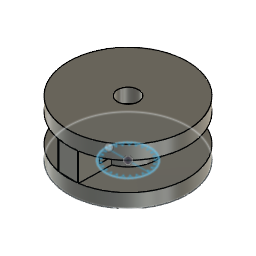
carrete servomotor (Autodesk Fusion 360 design; units mm, degrees)
part number: 2026-06-30-15-51-10-109
Autodesk Fusion 360 part; units mm, degrees
note: some values were not read from the file. Set by a fixed rule: which sketch regions a step uses.
sketch "Boceto1" plane through (0, 0, 0) normal (0, 0, 1) x (1, 0, 0)
  circle A0 centre (0, 0) radius 8.5
  line L0 (-3.15, 0) -> (3.15, 0)
  line L1 (-3.15, 0) -> (-2.6985, 0.2148)
  line L2 (-2.6985, 0.2148) -> (-3.1103, 0.4984)
  line L3 (-3.1103, 0.4984) -> (-3.15, 0)
  arc A1 (-3.15, 0) -> (-3.1103, 0.4984) centre (0, 0) ccw
  line L4 (-2.6672, -0.463) -> (-3.1366, -0.2907)
  line L5 (-3.1366, -0.2907) -> (-3.051, -0.7834)
  line L6 (-3.051, -0.7834) -> (-2.6672, -0.463)
  line L7 (-2.4682, -1.1117) -> (-2.9657, -1.0616)
  line L8 (-2.9657, -1.0616) -> (-2.7604, -1.5175)
  line L9 (-2.7604, -1.5175) -> (-2.4682, -1.1117)
  line L10 (-2.1142, -1.6906) -> (-2.6085, -1.7658)
  line L11 (-2.6085, -1.7658) -> (-2.2963, -2.1563)
  line L12 (-2.2963, -2.1563) -> (-2.1142, -1.6906)
  line L13 (-1.6273, -2.1633) -> (-2.0874, -2.3591)
  line L14 (-2.0874, -2.3591) -> (-1.6879, -2.6596)
  line L15 (-1.6879, -2.6596) -> (-1.6273, -2.1633)
  line L16 (-1.0382, -2.5) -> (-1.4352, -2.8041)
  line L17 (-1.4352, -2.8041) -> (-0.9734, -2.9958)
  line L18 (-0.9734, -2.9958) -> (-1.0382, -2.5)
  line L19 (-0.3839, -2.6797) -> (-0.6927, -3.0729)
  line L20 (-0.6927, -3.0729) -> (-0.1978, -3.1438)
  line L21 (-0.1978, -3.1438) -> (-0.3839, -2.6797)
  line L22 (0.2946, -2.691) -> (0.0932, -3.1486)
  line L23 (0.0932, -3.1486) -> (0.5903, -3.0942)
  line L24 (0.5903, -3.0942) -> (0.2946, -2.691)
  line L25 (0.9546, -2.5332) -> (0.8733, -3.0265)
  line L26 (0.8733, -3.0265) -> (1.3412, -2.8502)
  line L27 (1.3412, -2.8502) -> (0.9546, -2.5332)
  line L28 (1.5546, -2.2162) -> (1.5985, -2.7142)
  line L29 (1.5985, -2.7142) -> (2.0079, -2.4271)
  line L30 (2.0079, -2.4271) -> (1.5546, -2.2162)
  line L31 (2.0569, -1.76) -> (2.2233, -2.2314)
  line L32 (2.2233, -2.2314) -> (2.5484, -1.8515)
  line L33 (2.5484, -1.8515) -> (2.0569, -1.76)
  line L34 (2.4299, -1.1931) -> (2.7084, -1.6084)
  line L35 (2.7084, -1.6084) -> (2.9288, -1.1596)
  line L36 (2.9288, -1.1596) -> (2.4299, -1.1931)
  line L37 (2.6503, -0.5514) -> (3.0233, -0.8843)
  line L38 (3.0233, -0.8843) -> (3.1252, -0.3948)
  line L39 (3.1252, -0.3948) -> (2.6503, -0.5514)
  line L40 (2.7042, 0.1251) -> (3.1483, -0.1047)
  line L41 (3.1483, -0.1047) -> (3.1252, 0.3948)
  line L42 (3.1252, 0.3948) -> (2.7042, 0.1251)
  line L43 (2.5881, 0.7936) -> (3.0754, 0.6816)
  line L44 (3.0754, 0.6816) -> (2.9288, 1.1596)
  line L45 (2.9288, 1.1596) -> (2.5881, 0.7936)
  line L46 (2.3094, 1.4123) -> (2.8093, 1.425)
  line L47 (2.8093, 1.425) -> (2.5484, 1.8515)
  line L48 (2.5484, 1.8515) -> (2.3094, 1.4123)
  line L49 (1.8856, 1.9423) -> (2.3666, 2.0788)
  line L50 (2.3666, 2.0788) -> (2.0079, 2.4271)
  line L51 (2.0079, 2.4271) -> (1.8856, 1.9423)
  line L52 (1.3434, 2.3502) -> (1.7753, 2.6021)
  line L53 (1.7753, 2.6021) -> (1.3412, 2.8502)
  line L54 (1.3412, 2.8502) -> (1.3434, 2.3502)
  line L55 (0.7167, 2.6105) -> (1.0724, 2.9618)
  line L56 (1.0724, 2.9618) -> (0.5903, 3.0942)
  line L57 (0.5903, 3.0942) -> (0.7167, 2.6105)
  line L58 (0.045, 2.7067) -> (0.3021, 3.1355)
  line L59 (0.3021, 3.1355) -> (-0.1978, 3.1438)
  line L60 (-0.1978, 3.1438) -> (0.045, 2.7067)
  line L61 (-0.6296, 2.6328) -> (-0.4871, 3.1121)
  line L62 (-0.4871, 3.1121) -> (-0.9734, 2.9958)
  line L63 (-0.9734, 2.9958) -> (-0.6296, 2.6328)
  line L64 (-1.2645, 2.3935) -> (-1.2458, 2.8932)
  line L65 (-1.2458, 2.8932) -> (-1.6879, 2.6596)
  line L66 (-1.6879, 2.6596) -> (-1.2645, 2.3935)
  line L67 (-1.8201, 2.0039) -> (-1.9261, 2.4925)
  line L68 (-1.9261, 2.4925) -> (-2.2963, 2.1563)
  line L69 (-2.2963, 2.1563) -> (-1.8201, 2.0039)
  line L70 (-2.2612, 1.4883) -> (-2.4855, 1.9352)
  line L71 (-2.4855, 1.9352) -> (-2.7604, 1.5175)
  line L72 (-2.7604, 1.5175) -> (-2.2612, 1.4883)
  line L73 (-2.5603, 0.8792) -> (-2.8886, 1.2563)
  line L74 (-2.8886, 1.2563) -> (-3.051, 0.7834)
  line L75 (-3.051, 0.7834) -> (-2.5603, 0.8792)
  point P0 (-2.9863, 0.2378)
  dimension "d1" = 6.3
  dimension "d2" = 17
  dimension "d28" = 0.5
  dimension "d29" = 0.433
  dimension "d31" = 360
  constraint coincident A0.centre A1.centre
  constraint coincident L0.end A1
  constraint horizontal L0
  measures "d1" diameter of A1
  measures "d2" diameter of A0
  measures "d28" distance of L0.start L2.end
  measures "d29" distance of L1.end L3
extrude "Extruir1" add sketch "Boceto1" along normal blind 8 contours A0 | A1 L5 | L0 A1 L41 | L0 A1 L41 | A1 L74 | A1 L38 | A1 L8 | A1 L44 | A1 L71 | A1 L35 | A1 L11 | A1 L47 | A1 L68 | A1 L32 | A1 L14 | A1 L50 | A1 L65 | A1 L29 | A1 L17 | A1 L53 | A1 L62 | A1 L26 | A1 L20 | A1 L56 | A1 L59 | A1 L23
ref_plane "PlanoDeObra1" through (0, 0, 2) normal (0, 0, 1) x (1, 0, 0)
sketch "Boceto2" plane through (0, 0, 2) normal (0, 0, 1) x (1, 0, 0)
  circle A0 centre (0, 0) radius 4
  circle A1 centre (0, 0) radius 8.5
  line L0 (-1.5806, -3.6745) -> (1.4194, -3.7397)
  line L1 (1.4194, -3.7397) -> (1.3176, -8.4227)
  line L2 (1.3176, -8.4227) -> (-1.6824, -8.3575)
  line L3 (-1.6824, -8.3575) -> (-1.5806, -3.6745)
  dimension "d6" = 8
  dimension "d7" = 17
  dimension "d20" = 3
  constraint coincident A0.centre A1.centre
  constraint concentric A0 A1
  constraint perpendicular L0 L1
  constraint parallel L0 L2
  constraint parallel L1 L3
  constraint coincident A0 L0.end
  constraint coincident A0 L0.start
  measures "d6" diameter of A0
  measures "d7" diameter of A1
  measures "d20" horizontal distance of L0.start L0.end
extrude "Extruir2" cut sketch "Boceto2" along normal blind 4 contours A0 A1 L1 L3 | A0 A1 L1 L2 L3 | A1 L2
sketch "Boceto3" plane through (0, 0, 8) normal (0, 0, 1) x (-1, 0, 0)
  circle A0 centre (0, 0) radius 8.5
  circle A1 centre (0, 0) radius 1.5
  circle A2 centre (4, -5) radius 1
  circle A3 centre (5, 4) radius 1
  circle A4 centre (-4, 5) radius 1
  circle A5 centre (-5, -4) radius 1
  arc A6 (2.7604, -1.5175) -> (2.8886, -1.2563) centre (0, 0) ccw
  line L0 (3.051, -0.7834) -> (2.8886, -1.2563)
  line L1 (2.7604, -1.5175) -> (2.4855, -1.9352)
  arc A7 (2.2963, -2.1563) -> (2.4855, -1.9352) centre (0, 0) ccw
  line L2 (2.2963, -2.1563) -> (1.9261, -2.4925)
  arc A8 (1.6879, -2.6596) -> (1.9261, -2.4925) centre (0, 0) ccw
  line L3 (1.6879, -2.6596) -> (1.2458, -2.8932)
  arc A9 (0.9734, -2.9958) -> (1.2458, -2.8932) centre (0, 0) ccw
  line L4 (0.9734, -2.9958) -> (0.4871, -3.1121)
  arc A10 (0.1978, -3.1438) -> (0.4871, -3.1121) centre (0, 0) ccw
  line L5 (0.1978, -3.1438) -> (-0.3021, -3.1355)
  arc A11 (-0.5903, -3.0942) -> (-0.3021, -3.1355) centre (0, 0) ccw
  line L6 (-0.5903, -3.0942) -> (-1.0724, -2.9618)
  arc A12 (-1.3412, -2.8502) -> (-1.0724, -2.9618) centre (0, 0) ccw
  line L7 (-1.3412, -2.8502) -> (-1.7753, -2.6021)
  arc A13 (-2.0079, -2.4271) -> (-1.7753, -2.6021) centre (0, 0) ccw
  line L8 (-2.0079, -2.4271) -> (-2.3666, -2.0788)
  arc A14 (-2.5484, -1.8515) -> (-2.3666, -2.0788) centre (0, 0) ccw
  line L9 (-2.5484, -1.8515) -> (-2.8093, -1.425)
  arc A15 (-2.9288, -1.1596) -> (-2.8093, -1.425) centre (0, 0) ccw
  line L10 (-2.9288, -1.1596) -> (-3.0754, -0.6816)
  arc A16 (-3.1252, -0.3948) -> (-3.0754, -0.6816) centre (0, 0) ccw
  line L11 (-3.1252, -0.3948) -> (-3.1483, 0.1047)
  arc A17 (-3.1252, 0.3948) -> (-3.1483, 0.1047) centre (0, 0) ccw
  line L12 (-3.1252, 0.3948) -> (-3.0233, 0.8843)
  arc A18 (-2.9288, 1.1596) -> (-3.0233, 0.8843) centre (0, 0) ccw
  line L13 (-2.9288, 1.1596) -> (-2.7084, 1.6084)
  arc A19 (-2.5484, 1.8515) -> (-2.7084, 1.6084) centre (0, 0) ccw
  line L14 (-2.5484, 1.8515) -> (-2.2233, 2.2314)
  arc A20 (-2.0079, 2.4271) -> (-2.2233, 2.2314) centre (0, 0) ccw
  line L15 (-2.0079, 2.4271) -> (-1.5985, 2.7142)
  arc A21 (-1.3412, 2.8502) -> (-1.5985, 2.7142) centre (0, 0) ccw
  line L16 (-1.3412, 2.8502) -> (-0.8733, 3.0265)
  arc A22 (-0.5903, 3.0942) -> (-0.8733, 3.0265) centre (0, 0) ccw
  line L17 (-0.5903, 3.0942) -> (-0.0932, 3.1486)
  arc A23 (0.1978, 3.1438) -> (-0.0932, 3.1486) centre (0, 0) ccw
  line L18 (0.1978, 3.1438) -> (0.6927, 3.0729)
  arc A24 (0.9734, 2.9958) -> (0.6927, 3.0729) centre (0, 0) ccw
  line L19 (0.9734, 2.9958) -> (1.4352, 2.8041)
  arc A25 (1.6879, 2.6596) -> (1.4352, 2.8041) centre (0, 0) ccw
  line L20 (1.6879, 2.6596) -> (2.0874, 2.3591)
  arc A26 (2.2963, 2.1563) -> (2.0874, 2.3591) centre (0, 0) ccw
  line L21 (2.2963, 2.1563) -> (2.6085, 1.7658)
  arc A27 (2.7604, 1.5175) -> (2.6085, 1.7658) centre (0, 0) ccw
  line L22 (2.7604, 1.5175) -> (2.9657, 1.0616)
  arc A28 (3.051, 0.7834) -> (2.9657, 1.0616) centre (0, 0) ccw
  line L23 (3.051, 0.7834) -> (3.1366, 0.2907)
  arc A29 (3.15, 0) -> (3.1366, 0.2907) centre (0, 0) ccw
  line L24 (3.15, 0) -> (3.1103, -0.4984)
  arc A30 (3.051, -0.7834) -> (3.1103, -0.4984) centre (0, 0) ccw
  dimension "d10" = 3
  dimension "d13" = 2
  dimension "d15" = 360
  measures "d10" diameter of A1
  measures "d13" diameter of A2
extrude "Extruir6" add sketch "Boceto2" along normal blind 4 contours A0 A1 L1 L2 L3
sketch "Boceto5" plane through (1.5, -0.0326, 0) normal (0.999764, -0.02173, 0) x (0.02173, 0.999764, 0)
  line L0 (-8.3665, 2) -> (-3.708, 2)
  line L1 (-3.708, 2) -> (-3.708, 6)
  line L2 (-3.708, 6) -> (-8.3665, 6)
  line L3 (-8.3665, 6) -> (-8.3665, 2)
  line L4 (-8.3665, 6) -> (-8.3665, 2)
  line L5 (-8.3665, 6) -> (-3.708, 6)
  line L6 (-3.3921, 3) -> (-5.3921, 3)
  line L7 (-5.3921, 3) -> (-5.3921, 5)
  line L8 (-5.3921, 5) -> (-3.3921, 5)
  line L9 (-3.3921, 5) -> (-3.3921, 3)
  line L10 (-3.3921, 3) -> (-5.3921, 5) construction
  line L11 (-5.3921, 3) -> (-3.3921, 5) construction
  line L12 (-8.3921, 2) -> (-8.3921, 6)
  point P0 (-4.3921, 4)
  dimension "d23" = 2
  dimension "d24" = 2
  dimension "d25" = 3
  constraint coincident L2.end L3.start
  constraint coincident L0.start L3.end
  constraint coincident L1.end L2.start
  constraint horizontal L6
  constraint perpendicular L6 L7
  constraint parallel L6 L8
  constraint parallel L7 L9
  constraint coincident L10 P0
  constraint coincident L11 P0
  measures "d23" distance of L7.end L8.end
  measures "d24" distance of L6.end L7.end
  measures "d25" distance of L7 L12
extrude "Extruir7" cut sketch "Boceto5" along normal mid plane 7 contours L1 L6 L7 L8 | L1 L6 L8 L9
extrude "Extruir9" add sketch "Boceto3" against normal blind 2 contours A6 L0 L1 A7 L2 A8 L3 A9 L4 A10 L5 A11 L6 A12 L7 A13 L8 A14 L9 A15 L10 A16 L11 A17 L12 A18 L13 A19 L14 A20 L15 A21 L16 A22 L17 A23 L18 A24 L19 A25 L20 A26 L21 A27 L22 A28 L23 A29 L24 A30
extrude "Extruir10" add sketch "Boceto1" along normal blind 6 contours L1 L2 L3 | L0 L40 L41 L42 | L0 L40 L41 | L4 L5 L6 | L73 L74 L75 | L37 L38 L39 | L7 L8 L9 | L43 L44 L45 | L70 L71 L72 | L34 L35 L36 | L10 L11 L12 | L46 L47 L48 | L67 L68 L69 | L31 L32 L33 | L13 L14 L15 | L49 L50 L51 | L64 L65 L66 | L28 L29 L30 | L16 L17 L18 | L52 L53 L54 | L61 L62 L63 | L25 L26 L27 | L19 L20 L21 | L55 L56 L57 | L58 L59 L60 | L22 L23 L24
